Autodesk Fusion 360 part; units mm, degrees
(part 2 of 4)
sketch "intraboard_to_walls" plane through (0, 0, 0) normal (0, 0, 1) x (1, 0, 0)
  line L0 (107.12, 0) -> (107.12, 230) construction
  line L1 (100, 230) -> (-100, 230)
  line L2 (72.32, 0) -> (72.32, 230) construction
  line L3 (77.92, 0) -> (77.92, 230) construction
  line L4 (-79.68, 0) -> (-79.68, 230) construction
  line L5 (-85.28, 230) -> (-85.28, 0) construction
  line L6 (-107.12, 0) -> (-107.12, 230) construction
  line L7 (107.32, 0) -> (107.12, 0) construction
  line L8 (-107.32, 0) -> (-107.12, 0) construction
  line L9 (100, 202.925) -> (100, 197.075) construction
  line L10 (100, 157.075) -> (100, 162.925) construction
  line L11 (100, 117.075) -> (100, 122.925) construction
  line L12 (100, 77.075) -> (100, 82.925) construction
  line L13 (100, 37.075) -> (100, 42.925) construction
  line L14 (107.12, 42.925) -> (-107.12, 42.925) construction
  line L15 (107.12, 37.075) -> (-107.12, 37.075) construction
  line L16 (107.12, 77.075) -> (-107.12, 77.075) construction
  line L17 (107.12, 82.925) -> (-107.12, 82.925) construction
  line L18 (107.12, 117.075) -> (-107.12, 117.075) construction
  line L19 (107.12, 122.925) -> (-107.12, 122.925) construction
  line L20 (107.12, 157.075) -> (-107.12, 157.075) construction
  line L21 (107.12, 162.925) -> (-107.12, 162.925) construction
  line L22 (107.12, 197.075) -> (-107.12, 197.075) construction
  line L23 (107.12, 202.925) -> (-107.12, 202.925) construction
  line L24 (107.12, 208.925) -> (-107.12, 208.925) construction
  line L25 (107.12, 31.075) -> (-107.12, 31.075) construction
  line L26 (107.12, 31.075) -> (107.12, 37.075) construction
  line L27 (107.12, 202.925) -> (107.12, 208.925) construction
  line L28 (72.32, 208.925) -> (72.32, 202.925)
  line L29 (72.32, 202.925) -> (77.92, 202.925)
  line L30 (77.92, 202.925) -> (77.92, 197.075)
  line L31 (77.92, 197.075) -> (72.32, 197.075)
  line L32 (72.32, 197.075) -> (72.32, 162.925)
  line L33 (72.32, 162.925) -> (77.92, 162.925)
  line L34 (77.92, 162.925) -> (77.92, 157.075)
  line L35 (72.32, 157.075) -> (77.92, 157.075)
  line L36 (72.32, 157.075) -> (72.32, 122.925)
  line L37 (72.32, 122.925) -> (77.92, 122.925)
  line L38 (77.92, 122.925) -> (77.92, 117.075)
  line L39 (72.32, 117.075) -> (77.92, 117.075)
  line L40 (72.32, 31.075) -> (72.32, 37.075)
  line L41 (72.32, 42.925) -> (72.32, 77.075)
  line L42 (72.32, 82.925) -> (72.32, 117.075)
  line L43 (72.32, 82.925) -> (77.92, 82.925)
  line L44 (77.92, 77.075) -> (77.92, 82.925)
  line L45 (77.92, 37.075) -> (77.92, 42.925)
  line L46 (72.32, 37.075) -> (77.92, 37.075)
  line L47 (77.92, 42.925) -> (72.32, 42.925)
  line L48 (72.32, 77.075) -> (77.92, 77.075)
  line L49 (-79.68, 31.075) -> (-79.68, 37.075)
  line L50 (-79.68, 42.925) -> (-79.68, 77.075)
  line L51 (-79.68, 82.925) -> (-79.68, 117.075)
  line L52 (-79.68, 208.925) -> (-79.68, 202.925)
  line L53 (-79.68, 197.075) -> (-79.68, 162.925)
  line L54 (-79.68, 157.075) -> (-79.68, 122.925)
  line L55 (-85.28, 197.075) -> (-85.28, 202.925)
  line L56 (-85.28, 157.075) -> (-85.28, 162.925)
  line L57 (-85.28, 122.925) -> (-85.28, 117.075)
  line L58 (-85.28, 82.925) -> (-85.28, 77.075)
  line L59 (-85.28, 37.075) -> (-85.28, 42.925)
  line L60 (-79.68, 37.075) -> (-85.28, 37.075)
  line L61 (-79.68, 42.925) -> (-85.28, 42.925)
  line L62 (-79.68, 77.075) -> (-85.28, 77.075)
  line L63 (-79.68, 82.925) -> (-85.28, 82.925)
  line L64 (-79.68, 117.075) -> (-85.28, 117.075)
  line L65 (-79.68, 122.925) -> (-85.28, 122.925)
  line L66 (-79.68, 157.075) -> (-85.28, 157.075)
  line L67 (-79.68, 162.925) -> (-85.28, 162.925)
  line L68 (-85.28, 202.925) -> (-79.68, 202.925)
  line L69 (-79.68, 197.075) -> (-85.28, 197.075)
  line L70 (-107.12, 120) -> (107.12, 120) construction
  line L71 (107.12, 112.5) -> (107.12, 127.5)
  line L72 (-107.12, 112.5) -> (-107.12, 127.5)
  line L73 (-79.68, 31.075) -> (-107.12, 31.075)
  line L74 (-107.12, 31.075) -> (-107.12, 49.075)
  line L75 (-79.68, 208.925) -> (-107.12, 208.925)
  line L76 (-107.12, 208.925) -> (-107.12, 190.925)
  line L77 (72.32, 208.925) -> (107.12, 208.925)
  line L78 (107.12, 208.925) -> (107.12, 190.925)
  line L79 (72.32, 31.075) -> (107.12, 31.075)
  line L80 (107.12, 31.075) -> (107.12, 49.075)
  line L81 (-85.28, 0) -> (-90.28, 0) construction
  line L82 (-90.28, 0) -> (-90.28, 230) construction
  line L83 (77.92, 0) -> (82.92, 0) construction
  line L84 (82.92, 0) -> (82.92, 230) construction
  line L85 (-107.12, 49.075) -> (-90.28, 49.075)
  line L86 (-107.12, 112.5) -> (-90.28, 112.5)
  line L87 (-90.28, 112.5) -> (-90.28, 49.075)
  line L88 (107.12, 49.075) -> (82.92, 49.075)
  line L89 (107.12, 112.5) -> (82.92, 112.5)
  line L90 (-107.12, 190.925) -> (-90.28, 190.925)
  line L91 (107.12, 190.925) -> (82.92, 190.925)
  line L92 (107.12, 127.5) -> (82.92, 127.5)
  line L93 (-107.12, 127.5) -> (-90.28, 127.5)
  line L94 (-90.28, 127.5) -> (-90.28, 190.925)
  line L95 (82.92, 49.075) -> (82.92, 112.5)
  line L96 (82.92, 127.5) -> (82.92, 190.925)
  line L97 (-79.68, 202.925) -> (-79.68, 197.075)
  line L98 (-79.68, 162.925) -> (-79.68, 157.075)
  line L99 (-79.68, 122.925) -> (-79.68, 117.075)
  line L100 (-79.68, 82.925) -> (-79.68, 77.075)
  line L101 (-79.68, 42.925) -> (-79.68, 37.075)
  line L102 (72.32, 37.075) -> (72.32, 42.925)
  line L103 (72.32, 77.075) -> (72.32, 82.925)
  line L104 (72.32, 117.075) -> (72.32, 122.925)
  line L105 (72.32, 157.075) -> (72.32, 162.925)
  line L106 (72.32, 197.075) -> (72.32, 202.925)
  point P0 (77.92, 0)
  point P1 (72.32, 0)
  point P2 (107.32, 0)
  point P3 (-107.32, 0)
  point P4 (-85.28, 0)
  point P5 (-79.68, 0)
  point P6 (100, 40)
  point P7 (100, 80)
  point P8 (100, 120)
  point P9 (100, 160)
  point P10 (100, 200)
  point P11 (107.12, 120)
  point P12 (-107.12, 120)
  dimension "d132" = 0.2
  dimension "d133" = 5.85
  dimension "d134" = 6
  dimension "d135" = 15
  dimension "d136" = 18
  dimension "d137" = 5
  constraint coincident L0.end L1
  constraint vertical L0
  constraint horizontal P2 L0.start
  constraint coincident P1 L2.start
  constraint coincident L1 L2.end
  constraint perpendicular L1 L2
  constraint coincident P0 L3.start
  constraint coincident L1 L3.end
  constraint perpendicular L1 L3
  constraint coincident P5 L4.start
  constraint coincident L1 L4.end
  constraint perpendicular L1 L4
  constraint coincident L1 L5.start
  constraint coincident P4 L5.end
  constraint vertical L5
  constraint coincident L1 L6.end
  constraint horizontal P3 L6.start
  constraint coincident P2 L7.start
  constraint coincident P3 L8.start
  constraint equal L7 L8
  constraint vertical L6
  constraint parallel L0 L9
  constraint midpoint P10 L9
  constraint parallel L3 L10
  constraint vertical L11
  constraint vertical L12
  constraint vertical L13
  constraint equal L12 L13
  constraint equal L11 L12
  constraint equal L10 L11
  constraint equal L9 L10
  constraint midpoint P9 L10
  constraint midpoint P8 L11
  constraint midpoint P7 L12
  constraint midpoint P6 L13
  constraint coincident L0 L14.start
  constraint coincident L6 L14.end
  constraint perpendicular L6 L14
  constraint coincident L0 L15.start
  constraint coincident L6 L15.end
  constraint perpendicular L6 L15
  constraint coincident L0 L16.start
  constraint coincident L6 L16.end
  constraint perpendicular L6 L16
  constraint coincident L0 L17.start
  constraint coincident L6 L17.end
  constraint perpendicular L6 L17
  constraint coincident L0 L18.start
  constraint coincident L6 L18.end
  constraint perpendicular L6 L18
  constraint coincident L0 L19.start
  constraint coincident L6 L19.end
  constraint perpendicular L6 L19
  constraint coincident L0 L20.start
  constraint coincident L6 L20.end
  constraint perpendicular L6 L20
  constraint coincident L6 L21.end
  constraint perpendicular L6 L21
  constraint coincident L0 L22.start
  constraint coincident L6 L22.end
  constraint perpendicular L6 L22
  constraint coincident L0 L23.start
  constraint coincident L6 L23.end
  constraint perpendicular L6 L23
  constraint coincident L13.start L15
  constraint coincident L13.end L14
  constraint coincident L12.start L16
  constraint coincident L12.end L17
  constraint coincident L11.start L18
  constraint coincident L11.end L19
  constraint coincident L10.start L20
  constraint coincident L10.end L21
  constraint coincident L9.end L22
  constraint coincident L9.start L23
  constraint coincident L0 L24.start
  constraint coincident L6 L24.end
  constraint perpendicular L6 L24
  constraint coincident L6 L25.end
  constraint perpendicular L6 L25
  constraint coincident L0 L25.start
  constraint perpendicular L15 L26
  constraint equal L26 L27
  constraint coincident L24 L28.start
  constraint coincident L2 L28.start
  constraint coincident L23 L28.end
  constraint coincident L2 L28.end
  constraint coincident L23 L29.end
  constraint coincident L3 L29.end
  constraint coincident L22 L30.end
  constraint coincident L3 L30.end
  constraint coincident L2 L31.end
  constraint coincident L22 L31.end
  constraint coincident L2 L32.end
  constraint coincident L21 L32.end
  constraint coincident L3 L33.end
  constraint coincident L21 L33.end
  constraint coincident L20 L34.end
  constraint coincident L3 L34.end
  constraint coincident L20 L35.start
  constraint coincident L2 L35.start
  constraint coincident L19 L36.end
  constraint coincident L2 L36.end
  constraint coincident L19 L37.end
  constraint coincident L3 L37.end
  constraint coincident L3 L38.end
  constraint coincident L18 L38.end
  constraint coincident L18 L39.start
  constraint perpendicular L38 L39
  constraint coincident L25 L40.start
  constraint coincident L2 L40.start
  constraint coincident L15 L40.end
  constraint coincident L2 L40.end
  constraint coincident L14 L41.start
  constraint coincident L2 L41.start
  constraint coincident L16 L41.end
  constraint coincident L2 L41.end
  constraint coincident L17 L42.start
  constraint coincident L2 L42.start
  constraint perpendicular L18 L42
  constraint coincident L17 L43.end
  constraint coincident L3 L43.end
  constraint coincident L16 L44.start
  constraint coincident L3 L44.start
  constraint coincident L15 L45.start
  constraint coincident L3 L45.start
  constraint coincident L14 L45.end
  constraint coincident L3 L45.end
  constraint coincident L4 L49.start
  constraint coincident L25 L49.start
  constraint coincident L15 L49.end
  constraint coincident L4 L49.end
  constraint coincident L14 L50.start
  constraint coincident L4 L50.start
  constraint coincident L4 L50.end
  constraint coincident L16 L50.end
  constraint coincident L4 L51.start
  constraint coincident L17 L51.start
  constraint coincident L4 L51.end
  constraint coincident L18 L51.end
  constraint coincident L24 L52.start
  constraint coincident L4 L52.start
  constraint coincident L4 L52.end
  constraint coincident L23 L52.end
  constraint coincident L4 L53.start
  constraint coincident L22 L53.start
  constraint coincident L4 L53.end
  constraint coincident L21 L53.end
  constraint coincident L20 L54.start
  constraint coincident L4 L54.start
  constraint coincident L19 L54.end
  constraint coincident L4 L54.end
  constraint coincident L22 L55.start
  constraint coincident L5 L55.start
  constraint coincident L23 L55.end
  constraint coincident L5 L55.end
  constraint coincident L20 L56.start
  constraint coincident L5 L56.start
  constraint coincident L21 L56.end
  constraint coincident L5 L56.end
  constraint coincident L19 L57.start
  constraint coincident L5 L57.start
  constraint coincident L5 L57.end
  constraint coincident L18 L57.end
  constraint coincident L17 L58.start
  constraint coincident L5 L58.start
  constraint coincident L16 L58.end
  constraint coincident L5 L58.end
  constraint coincident L15 L59.start
  constraint coincident L5 L59.start
  constraint coincident L14 L59.end
  constraint coincident L5 L59.end
  constraint coincident L0 P11
  constraint coincident L6 P12
  constraint coincident P12 L70.start
  constraint coincident P11 L70.end
  constraint horizontal L70
  constraint coincident P8 L70
  constraint perpendicular L70 L71
  constraint midpoint P11 L71
  constraint coincident L0 L21.start
  constraint parallel L6 L72
  constraint equal L71 L72
  constraint midpoint P12 L72
  constraint coincident L6 L74.end
  constraint coincident L6 L76.end
  constraint coincident L0 L78.end
  constraint coincident L0 L80.end
  constraint equal L74 L80
  constraint equal L74 L76
  constraint equal L78 L80
  constraint perpendicular L5 L81
  constraint coincident L1 L82.end
  constraint perpendicular L1 L82
  constraint perpendicular L3 L83
  constraint coincident L1 L84.end
  constraint perpendicular L1 L84
  constraint equal L81 L83
  constraint coincident L82 L85.end
  constraint perpendicular L82 L85
  constraint coincident L82 L86.end
  constraint perpendicular L82 L86
  constraint coincident L84 L88.end
  constraint perpendicular L84 L88
  constraint coincident L84 L89.end
  constraint perpendicular L84 L89
  constraint coincident L82 L90.end
  constraint perpendicular L82 L90
  constraint coincident L84 L91.end
  constraint perpendicular L84 L91
  constraint coincident L84 L92.end
  constraint perpendicular L84 L92
  constraint coincident L82 L93.end
  constraint perpendicular L82 L93
  measures "d132" distance of P2 L0
  measures "d133" distance of L9.start L9.end
  measures "d134" distance of L15.start L25.start
  measures "d135" distance of L71.start L71.end
  measures "d136" distance of L25.end L74.end
  measures "d137" distance of P4 L81.end
extrude "Extrude5" add sketch "intraboard_to_walls" along normal up to surface (25.6 mm away) from surface at 21.5 separate body contours L28 L29 L30 L31 L32 L33 L34 L35 L36 L37 L38 L39 L40 L41 L42 L43 L44 L45 L46 L47 L48 L71 L77 L78 L79 L80 L88 L89 L91 L92 L95 L96 makes body 7
extrude "Extrude6" add sketch "intraboard_to_walls" along normal up to surface (5 mm away) from surface at 42.1 contours L29 L30 L31 L106 | L33 L34 L35 L105 | L37 L38 L39 L104 | L43 L44 L48 L103 | L45 L46 L47 L102 bodies 7
extrude "Extrude7" add sketch "intraboard_to_walls" along normal up to surface (22.6 mm away) from surface at 21.5 separate body contours L49 L50 L51 L52 L53 L54 L55 L56 L57 L58 L59 L60 L61 L62 L63 L64 L65 L66 L67 L68 L69 L72 L73 L74 L75 L76 L85 L86 L87 L90 L93 L94 makes body 8
extrude "Extrude8" add sketch "intraboard_to_walls" along normal up to surface (2 mm away) from surface at 42.1 contours L59 L60 L61 L101 | L58 L62 L63 L100 | L57 L64 L65 L99 | L56 L66 L67 L98 | L55 L68 L69 L97 bodies 8
extrude "Extrude9" add sketch "left side panel" along normal up to surface (5.36 mm away) from surface at 107.32 separate body makes body 9
ref_plane "WorkPlane1" through (-107.32, 0, 0) normal (1, 0, 0) x (0, 1, 0)
sketch "right side panel" plane through (-107.32, 0, 0) normal (1, 0, 0) x (0, 0, -1)
  line L0 (-105.5, 215.5) -> (105.5, 215.5)
  line L1 (105.5, 215.5) -> (105.5, 4.5)
  line L2 (-105.5, 4.5) -> (-105.5, 215.5)
  line L3 (105.5, 4.5) -> (-105.5, 4.5)
  line L4 (-21.5, 31.075) -> (-44.1, 31.075)
  line L5 (-44.1, 31.075) -> (-44.1, 49.075)
  line L6 (-44.1, 49.075) -> (-21.5, 49.075)
  line L7 (-21.5, 49.075) -> (-21.5, 31.075)
  line L8 (-21.5, 127.5) -> (-44.1, 127.5)
  line L9 (-44.1, 127.5) -> (-44.1, 112.5)
  line L10 (-44.1, 112.5) -> (-21.5, 112.5)
  line L11 (-21.5, 112.5) -> (-21.5, 127.5)
  line L12 (-21.5, 208.925) -> (-44.1, 208.925)
  line L13 (-44.1, 208.925) -> (-44.1, 190.925)
  line L14 (-44.1, 190.925) -> (-21.5, 190.925)
  line L15 (-21.5, 190.925) -> (-21.5, 208.925)
  line L16 (105.5, 215.5) -> (100, 215.5) construction
  line L17 (100, 215.5) -> (100, 210) construction
  line L18 (100, 210) -> (105.5, 210) construction
  line L19 (105.5, 210) -> (105.5, 215.5) construction
  line L20 (-105.5, 4.5) -> (-100, 4.5) construction
  line L21 (-100, 4.5) -> (-100, 10) construction
  line L22 (-100, 10) -> (-105.5, 10) construction
  line L23 (-105.5, 10) -> (-105.5, 4.5) construction
  line L24 (100, 210) -> (-100, 210) construction
  line L25 (-100, 210) -> (-100, 10) construction
  line L26 (-100, 10) -> (100, 10) construction
  line L27 (100, 10) -> (100, 210) construction
  line L28 (-100, 10) -> (-85, 10) construction
  line L29 (-85, 10) -> (-85, 25) construction
  line L30 (-85, 25) -> (-100, 25) construction
  line L31 (-100, 25) -> (-100, 10) construction
  line L32 (-73, 25) -> (-79, 35.3923) construction
  line L33 (-79, 35.3923) -> (-85, 25) construction
  line L34 (-85, 25) -> (-73, 25) construction
  line L35 (-79, 35.3923) -> (-73, 45.7846) construction
  line L36 (-73, 45.7846) -> (-85, 45.7846) construction
  line L37 (-85, 45.7846) -> (-79, 35.3923) construction
  line L38 (-100, 10) -> (-95, 10) construction
  line L39 (-95, 10) -> (-95, 15) construction
  line L40 (-95, 15) -> (-100, 15) construction
  line L41 (-100, 15) -> (-100, 10) construction
  line L42 (-100, 210) -> (-95, 210) construction
  line L43 (-95, 210) -> (-95, 205) construction
  line L44 (-95, 205) -> (-100, 205) construction
  line L45 (-100, 205) -> (-100, 210) construction
  line L46 (-95, 15) -> (-15, 15) construction
  line L47 (-15, 15) -> (-15, 205) construction
  line L48 (-15, 205) -> (-95, 205) construction
  line L49 (-95, 205) -> (-95, 15) construction
  line L50 (-79, 35.3923) -> (-91, 35.3923) construction
  line L51 (-21.5, 208.925) -> (-44.1, 190.925) construction
  line L52 (-21.5, 127.5) -> (-44.1, 112.5) construction
  line L53 (-21.5, 49.075) -> (-44.1, 31.075) construction
  arc A0 (-32.4011, 44.6367) -> (-33.1989, 44.6367) centre (-32.8, 44.667) ccw
  line L54 (-32.8, 40.075) -> (-32.8, 44.867) construction
  line L55 (-36.95, 42.0104) -> (-36.95, 38.1396)
  line L56 (-36.5511, 37.4487) -> (-33.1989, 35.5133)
  line L57 (-28.65, 38.1396) -> (-28.65, 42.0104)
  arc A1 (-33.1989, 35.5133) -> (-32.4011, 35.5133) centre (-32.8, 35.483) ccw
  line L58 (-28.65, 37.679) -> (-28.65, 42.471) construction
  line L59 (-32.4011, 35.5133) -> (-29.0489, 37.4487)
  arc A2 (-28.65, 42.0104) -> (-29.0489, 42.7013) centre (-28.8232, 42.371) ccw
  line L60 (-36.95, 42.471) -> (-36.95, 37.679) construction
  line L61 (-28.65, 42.471) -> (-32.8, 44.867) construction
  circle A3 centre (-32.8, 44.667) radius 0.4 construction
  line L62 (-33.1989, 44.6367) -> (-36.5511, 42.7013)
  line L63 (-29.0489, 42.7013) -> (-32.4011, 44.6367)
  arc A4 (-36.95, 38.1396) -> (-36.5511, 37.4487) centre (-36.7768, 37.779) ccw
  line L64 (-32.8, 44.867) -> (-36.95, 42.471) construction
  arc A5 (-36.5511, 42.7013) -> (-36.95, 42.0104) centre (-36.7768, 42.371) ccw
  line L65 (-36.95, 37.679) -> (-32.8, 35.283) construction
  line L66 (-32.8, 35.283) -> (-28.65, 37.679) construction
  arc A6 (-29.0489, 37.4487) -> (-28.65, 38.1396) centre (-28.8232, 37.779) ccw
  arc A7 (-33.1989, 115.4383) -> (-32.4011, 115.4383) centre (-32.8, 115.408) ccw
  arc A8 (-32.4011, 124.5617) -> (-33.1989, 124.5617) centre (-32.8, 124.592) ccw
  line L67 (-29.0489, 122.6263) -> (-32.4011, 124.5617)
  line L68 (-28.65, 122.396) -> (-32.8, 124.792) construction
  line L69 (-28.65, 117.604) -> (-28.65, 122.396) construction
  line L70 (-32.8, 124.792) -> (-36.95, 122.396) construction
  line L71 (-32.8, 115.208) -> (-28.65, 117.604) construction
  line L72 (-33.1989, 124.5617) -> (-36.5511, 122.6263)
  line L73 (-32.8, 120) -> (-32.8, 124.792) construction
  line L74 (-36.95, 117.604) -> (-32.8, 115.208) construction
  line L75 (-32.4011, 115.4383) -> (-29.0489, 117.3737)
  line L76 (-28.65, 118.0646) -> (-28.65, 121.9354)
  arc A9 (-28.65, 121.9354) -> (-29.0489, 122.6263) centre (-28.8232, 122.296) ccw
  arc A10 (-36.5511, 122.6263) -> (-36.95, 121.9354) centre (-36.7768, 122.296) ccw
  line L77 (-36.95, 122.396) -> (-36.95, 117.604) construction
  circle A11 centre (-32.8, 124.592) radius 0.4 construction
  arc A12 (-29.0489, 117.3737) -> (-28.65, 118.0646) centre (-28.8232, 117.704) ccw
  line L78 (-36.95, 121.9354) -> (-36.95, 118.0646)
  arc A13 (-36.95, 118.0646) -> (-36.5511, 117.3737) centre (-36.7768, 117.704) ccw
  line L79 (-36.5511, 117.3737) -> (-33.1989, 115.4383)
  arc A14 (-33.1989, 195.3633) -> (-32.4011, 195.3633) centre (-32.8, 195.333) ccw
  arc A15 (-32.4011, 204.4867) -> (-33.1989, 204.4867) centre (-32.8, 204.517) ccw
  line L80 (-29.0489, 202.5513) -> (-32.4011, 204.4867)
  line L81 (-28.65, 202.321) -> (-32.8, 204.717) construction
  line L82 (-28.65, 197.529) -> (-28.65, 202.321) construction
  line L83 (-32.8, 204.717) -> (-36.95, 202.321) construction
  line L84 (-32.8, 195.133) -> (-28.65, 197.529) construction
  line L85 (-33.1989, 204.4867) -> (-36.5511, 202.5513)
  line L86 (-32.8, 199.925) -> (-32.8, 204.717) construction
  line L87 (-36.95, 197.529) -> (-32.8, 195.133) construction
  line L88 (-32.4011, 195.3633) -> (-29.0489, 197.2987)
  line L89 (-28.65, 197.9896) -> (-28.65, 201.8604)
  arc A16 (-28.65, 201.8604) -> (-29.0489, 202.5513) centre (-28.8232, 202.221) ccw
  arc A17 (-36.5511, 202.5513) -> (-36.95, 201.8604) centre (-36.7768, 202.221) ccw
  line L90 (-36.95, 202.321) -> (-36.95, 197.529) construction
  circle A18 centre (-32.8, 204.517) radius 0.4 construction
  arc A19 (-29.0489, 197.2987) -> (-28.65, 197.9896) centre (-28.8232, 197.629) ccw
  line L91 (-36.95, 201.8604) -> (-36.95, 197.9896)
  arc A20 (-36.95, 197.9896) -> (-36.5511, 197.2987) centre (-36.7768, 197.629) ccw
  line L92 (-36.5511, 197.2987) -> (-33.1989, 195.3633)
  point P0 (-21.5, 0)
  point P1 (-44.1, 0)
  point P2 (0, 31.075)
  point P3 (0, 49.075)
  point P4 (0, 112.5)
  point P5 (0, 127.5)
  point P6 (0, 190.925)
  point P7 (0, 208.925)
  point P8 (-79, 28.4641)
  point P9 (-61, 25)
  point P10 (-49, 25)
  point P11 (-37, 25)
  point P12 (-25, 25)
  point P13 (-85, 45.785)
  point P14 (-73, 45.785)
  point P15 (-61, 45.785)
  point P16 (-49, 45.785)
  point P17 (-85, 66.57)
  point P18 (-73, 66.57)
  point P19 (-61, 66.57)
  point P20 (-49, 66.57)
  point P21 (-37, 66.57)
  point P22 (-25, 66.57)
  point P23 (-85, 87.355)
  point P24 (-73, 87.355)
  point P25 (-61, 87.355)
  point P26 (-49, 87.355)
  point P27 (-37, 87.355)
  point P28 (-25, 87.355)
  point P29 (-85, 108.14)
  point P30 (-73, 108.14)
  point P31 (-61, 108.14)
  point P32 (-49, 108.14)
  point P33 (-85, 128.925)
  point P34 (-73, 128.925)
  point P35 (-61, 128.925)
  point P36 (-49, 128.925)
  point P37 (-85, 149.71)
  point P38 (-73, 149.71)
  point P39 (-61, 149.71)
  point P40 (-49, 149.71)
  point P41 (-37, 149.71)
  point P42 (-25, 149.71)
  point P43 (-85, 170.495)
  point P44 (-73, 170.495)
  point P45 (-61, 170.495)
  point P46 (-49, 170.495)
  point P47 (-37, 170.495)
  point P48 (-25, 170.495)
  point P49 (-85, 191.28)
  point P50 (-73, 191.28)
  point P51 (-61, 191.28)
  point P52 (-49, 191.28)
  point P53 (-67, 35.3923)
  point P54 (-55, 35.3923)
  point P55 (-91, 56.1773)
  point P56 (-79, 56.1773)
  point P57 (-67, 56.1773)
  point P58 (-55, 56.1773)
  point P59 (-43, 56.1773)
  point P60 (-31, 56.1773)
  point P61 (-19, 56.1773)
  point P62 (-91, 76.9623)
  point P63 (-79, 76.9623)
  point P64 (-67, 76.9623)
  point P65 (-55, 76.9623)
  point P66 (-43, 76.9623)
  point P67 (-31, 76.9623)
  point P68 (-19, 76.9623)
  point P69 (-91, 97.7473)
  point P70 (-79, 97.7473)
  point P71 (-67, 97.7473)
  point P72 (-55, 97.7473)
  point P73 (-43, 97.7473)
  point P74 (-31, 97.7473)
  point P75 (-19, 97.7473)
  point P76 (-91, 118.5323)
  point P77 (-79, 118.5323)
  point P78 (-67, 118.5323)
  point P79 (-55, 118.5323)
  point P80 (-91, 139.3173)
  point P81 (-79, 139.3173)
  point P82 (-67, 139.3173)
  point P83 (-55, 139.3173)
  point P84 (-43, 139.3173)
  point P85 (-31, 139.3173)
  point P86 (-19, 139.3173)
  point P87 (-91, 160.1023)
  point P88 (-79, 160.1023)
  point P89 (-67, 160.1023)
  point P90 (-55, 160.1023)
  point P91 (-43, 160.1023)
  point P92 (-31, 160.1023)
  point P93 (-19, 160.1023)
  point P94 (-91, 180.8873)
  point P95 (-79, 180.8873)
  point P96 (-67, 180.8873)
  point P97 (-55, 180.8873)
  point P98 (-43, 180.8873)
  point P99 (-31, 180.8873)
  point P100 (-19, 180.8873)
  point P101 (-91, 201.6723)
  point P102 (-79, 201.6723)
  point P103 (-67, 201.6723)
  point P104 (-55, 201.6723)
  point P105 (-32.8, 40.075)
  point P106 (-32.8, 120)
  point P107 (-32.8, 199.925)
  point P108 (-32.8, 40.075)
  point P109 (-32.8, 40.075)
  point P110 (-32.8, 40.075)
  point P111 (-32.8, 40.075)
  point P112 (-32.8, 120)
  point P113 (-32.8, 120)
  point P114 (-32.8, 120)
  point P115 (-32.8, 120)
  point P116 (-32.8, 120)
  point P117 (-32.8, 199.925)
  point P118 (-32.8, 199.925)
  point P119 (-32.8, 199.925)
  point P120 (-32.8, 199.925)
  point P121 (-32.8, 199.925)
  dimension "d154" = 5.5
  dimension "d156" = 15
  dimension "d157" = 15
  dimension "d158" = 12
  dimension "d159" = 12
  dimension "d160" = 20.7846
  dimension "d161" = 5
  dimension "d162" = 5
  dimension "d163" = 80
  dimension "d166" = 12
  dimension "d167" = 20.785
  dimension "d171" = 12
  dimension "d172" = 20.785
  dimension "d261" = 360
  dimension "d263" = 360
  dimension "d264" = 4.15
  dimension "d265" = 0.8
  dimension "d266" = 0.2
  dimension "d268" = 360
  dimension "d270" = 360
  dimension "d271" = 4.15
  dimension "d272" = 0.8
  dimension "d273" = 0.2
  dimension "d275" = 360
  dimension "d277" = 360
  dimension "d278" = 4.15
  dimension "d279" = 0.8
  dimension "d280" = 0.2
  constraint horizontal L4
  constraint vertical L5
  constraint horizontal L6
  constraint vertical L7
  constraint horizontal L8
  constraint vertical L9
  constraint horizontal L10
  constraint vertical L11
  constraint horizontal L12
  constraint vertical L13
  constraint horizontal L14
  constraint vertical L15
  constraint coincident P7 L12
  constraint coincident P6 L14
  constraint coincident P5 L8
  constraint coincident P4 L10
  constraint coincident P3 L6
  constraint coincident P2 L4
  constraint coincident P0 L7
  constraint coincident P1 L5
  constraint coincident P0 L11
  constraint coincident P1 L9
  constraint coincident P0 L15
  constraint coincident P1 L13
  constraint horizontal L16
  constraint vertical L17
  constraint horizontal L18
  constraint vertical L19
  constraint coincident L0.end L1.start
  constraint equal L17 L18
  constraint horizontal L20
  constraint vertical L21
  constraint horizontal L22
  constraint vertical L23
  constraint coincident L2.start L3.end
  constraint equal L21 L22
  constraint equal L18 L22
  constraint horizontal L24
  constraint vertical L25
  constraint horizontal L26
  constraint vertical L27
  constraint horizontal L28
  constraint vertical L29
  constraint horizontal L30
  constraint vertical L31
  constraint coincident L29.end L30.start
  constraint horizontal L34
  constraint parallel L33 L35
  constraint horizontal L36
  constraint parallel L32 L37
  constraint horizontal L38
  constraint vertical L39
  constraint horizontal L40
  constraint vertical L41
  constraint horizontal L42
  constraint vertical L43
  constraint horizontal L44
  constraint vertical L45
  constraint equal L43 L44
  constraint equal L40 L44
  constraint horizontal L46
  constraint vertical L47
  constraint horizontal L48
  constraint vertical L49
  constraint coincident L43.end L44.start
  constraint horizontal L50
  constraint equal L34 L50
  constraint midpoint L53 P111
  constraint midpoint L52 P116
  constraint midpoint L51 P121
  constraint coincident P111 P110
  constraint vertical L60
  constraint coincident A0.centre L54
  constraint coincident A0.end L64
  constraint coincident A0.start L61
  constraint coincident A0.start A3
  constraint coincident A0.centre A3.centre
  constraint coincident P116 P115
  constraint vertical L77
  constraint coincident A8.centre L73
  constraint coincident A8.end L70
  constraint coincident A8.start L68
  constraint coincident A8.start A11
  constraint coincident A8.centre A11.centre
  constraint coincident P121 P120
  constraint vertical L90
  constraint coincident A15.centre L86
  constraint coincident A15.end L83
  constraint coincident A15.start L81
  constraint coincident A15.start A18
  constraint coincident A15.centre A18.centre
  measures "d154" distance of L0.end L18.end
  measures "d156" distance of L21.end L28.end
  measures "d157" distance of L21.end L30.end
  measures "d158" distance of L32.start L29.end
  measures "d159" distance of L32.end L35.end
  measures "d160" distance of L29.end L36.end
  measures "d161" distance of L21.end L38.end
  measures "d162" distance of L21.end L40.end
  measures "d163" distance of L39.end L46.end
  measures "d264" distance of P111 L60
  measures "d265" diameter of A3
  measures "d266" distance of L54.end A0.centre
  measures "d271" distance of P116 L77
  measures "d272" diameter of A11
  measures "d273" distance of A8.centre L68.end
  measures "d278" distance of P121 L90
  measures "d279" diameter of A18
  measures "d280" distance of A15.centre L81.end
extrude "Extrude10" add sketch "right side panel" against normal up to surface (5.36 mm away) separate body contours L0 L1 L2 L3 | L4 L5 L6 L7 | L8 L9 L10 L11 | L12 L13 L14 L15 | A0 L55 L56 L57 A1 L59 A2 L62 L63 A4 A5 A6 | A7 A8 L67 L72 L75 L76 A9 A10 A12 L78 A13 L79 | A14 A15 L80 L85 L88 L89 A16 A17 A19 L91 A20 L92 makes body 10
hole "Hole1" at (-107.32, 191.28, 61) at (-107.32, 191.28, 49) at (-107.32, 180.8873, 43) at (-107.32, 180.8873, 31) at (-107.32, 180.8873, 19) at (-107.32, 170.495, 25) at (-107.32, 160.1023, 19) at (-107.32, 149.71, 25) at (-107.32, 139.3173, 19) at (-107.32, 139.3173, 31) at (-107.32, 139.3173, 43) at (-107.32, 128.925, 49) at (-107.32, 118.5323, 55) at (-107.32, 108.14, 49) at (-107.32, 97.7473, 43) at (-107.32, 97.7473, 31) at (-107.32, 97.7473, 19) at (-107.32, 87.355, 25) at (-107.32, 87.355, 37) at (-107.32, 76.9623, 19) at (-107.32, 76.9623, 31) at (-107.32, 76.9623, 43) at (-107.32, 87.355, 49) at (-107.32, 56.1773, 19) at (-107.32, 66.57, 25) at (-107.32, 56.1773, 31) at (-107.32, 56.1773, 43) at (-107.32, 45.785, 49) at (-107.32, 35.3923, 55) at (-107.32, 25, 49) at (-107.32, 25, 37) at (-107.32, 25, 25) at (-107.32, 25, 61) at (-107.32, 35.3923, 67) at (-107.32, 45.785, 61) at (-107.32, 25, 73) at (-107.32, 25, 85) at (-107.32, 35.3923, 79) at (-107.32, 45.785, 85) at (-107.32, 45.785, 73) at (-107.32, 56.1773, 67) at (-107.32, 56.1773, 55) at (-107.32, 66.57, 49) at (-107.32, 66.57, 37) at (-107.32, 66.57, 61) at (-107.32, 76.9623, 55) at (-107.32, 76.9623, 67) at (-107.32, 66.57, 73) at (-107.32, 87.355, 61) at (-107.32, 56.1773, 79) at (-107.32, 66.57, 85) at (-107.32, 76.9623, 79) at (-107.32, 87.355, 85) at (-107.32, 87.355, 73) at (-107.32, 97.7473, 79) at (-107.32, 108.14, 85) at (-107.32, 118.5323, 79) at (-107.32, 128.925, 85) at (-107.32, 139.3173, 79) at (-107.32, 149.71, 85) at (-107.32, 160.1023, 79) at (-107.32, 160.1023, 67) at (-107.32, 160.1023, 55) at (-107.32, 160.1023, 43) at (-107.32, 160.1023, 31) at (-107.32, 149.71, 37) at (-107.32, 149.71, 49) at (-107.32, 149.71, 61) at (-107.32, 139.3173, 55) at (-107.32, 128.925, 61) at (-107.32, 108.14, 61) at (-107.32, 97.7473, 55) at (-107.32, 97.7473, 67) at (-107.32, 108.14, 73) at (-107.32, 118.5323, 67) at (-107.32, 128.925, 73) at (-107.32, 139.3173, 67) at (-107.32, 149.71, 73) at (-107.32, 170.495, 85) at (-107.32, 180.8873, 79) at (-107.32, 191.28, 85) at (-107.32, 191.28, 73) at (-107.32, 180.8873, 67) at (-107.32, 180.8873, 55) at (-107.32, 170.495, 37) at (-107.32, 170.495, 49) at (-107.32, 170.495, 61) at (-107.32, 170.495, 73) direction (-1, 0, 0) diameter 10 end up to surface (5.36 mm away) bodies 10
sketch "left_side_misc" plane through (0, 0, 0) normal (1, 0, 0) x (0, 0, -1)
  line L0 (-47.1, 208.925) -> (-47.1, 190.925) construction
  line L1 (-47.1, 190.925) -> (-21.5, 190.925) construction
  line L2 (-21.5, 190.925) -> (-21.5, 208.925) construction
  line L3 (-21.5, 208.925) -> (-47.1, 208.925) construction
  line L4 (-47.1, 127.5) -> (-47.1, 112.5) construction
  line L5 (-47.1, 112.5) -> (-21.5, 112.5) construction
  line L6 (-21.5, 112.5) -> (-21.5, 127.5) construction
  line L7 (-21.5, 127.5) -> (-47.1, 127.5) construction
  line L8 (-47.1, 49.075) -> (-47.1, 31.075) construction
  line L9 (-47.1, 31.075) -> (-21.5, 31.075) construction
  line L10 (-21.5, 31.075) -> (-21.5, 49.075) construction
  line L11 (-21.5, 49.075) -> (-47.1, 49.075) construction
  line L12 (-47.1, 208.925) -> (-21.5, 190.925) construction
  line L13 (-47.1, 127.5) -> (-21.5, 112.5) construction
  line L14 (-21.5, 31.075) -> (-47.1, 49.075) construction
  line L15 (-77, 45) -> (-51, 45)
  line L16 (-51, 45) -> (-51, 14)
  line L17 (-51, 14) -> (-77, 14)
  line L18 (-77, 14) -> (-77, 45)
  line L19 (-64, 14) -> (-64, 45) construction
  line L20 (-51, 29.5) -> (-77, 29.5) construction
  line L21 (-73.6, 41.5) -> (-54.4, 17.5) construction
  circle A0 centre (-64, 29.5) radius 11.6
  circle A1 centre (-73.6, 41.5) radius 1.1
  circle A2 centre (-54.4, 17.5) radius 1.1
  line L22 (-30.15, 122.396) -> (-34.3, 124.792) construction
  line L23 (-34.3, 124.792) -> (-38.45, 122.396) construction
  line L24 (-38.45, 122.396) -> (-38.45, 117.604) construction
  line L25 (-38.45, 117.604) -> (-34.3, 115.208) construction
  line L26 (-34.3, 115.208) -> (-30.15, 117.604) construction
  line L27 (-30.15, 117.604) -> (-30.15, 122.396) construction
  circle A3 centre (-34.3, 124.592) radius 0.4 construction
  circle A4 centre (-38.2768, 122.296) radius 0.4 construction
  circle A5 centre (-38.2768, 117.704) radius 0.4 construction
  circle A6 centre (-34.3, 115.408) radius 0.4 construction
  circle A7 centre (-30.3232, 117.704) radius 0.4 construction
  circle A8 centre (-30.3232, 122.296) radius 0.4 construction
  arc A9 (-33.9011, 124.5617) -> (-34.6989, 124.5617) centre (-34.3, 124.592) ccw
  arc A10 (-38.0511, 122.6263) -> (-38.45, 121.9354) centre (-38.2768, 122.296) ccw
  arc A11 (-38.45, 118.0646) -> (-38.0511, 117.3737) centre (-38.2768, 117.704) ccw
  arc A12 (-34.6989, 115.4383) -> (-33.9011, 115.4383) centre (-34.3, 115.408) ccw
  arc A13 (-30.5489, 117.3737) -> (-30.15, 118.0646) centre (-30.3232, 117.704) ccw
  arc A14 (-30.15, 121.9354) -> (-30.5489, 122.6263) centre (-30.3232, 122.296) ccw
  line L28 (-33.9011, 124.5617) -> (-30.5489, 122.6263)
  line L29 (-38.0511, 122.6263) -> (-34.6989, 124.5617)
  line L30 (-38.45, 118.0646) -> (-38.45, 121.9354)
  line L31 (-34.6989, 115.4383) -> (-38.0511, 117.3737)
  line L32 (-30.5489, 117.3737) -> (-33.9011, 115.4383)
  line L33 (-30.15, 121.9354) -> (-30.15, 118.0646)
  line L34 (-30.5489, 37.4487) -> (-33.9011, 35.5133)
  arc A15 (-30.5489, 37.4487) -> (-30.15, 38.1396) centre (-30.3232, 37.779) ccw
  circle A16 centre (-38.2768, 42.371) radius 0.4 construction
  arc A17 (-30.15, 42.0104) -> (-30.5489, 42.7013) centre (-30.3232, 42.371) ccw
  circle A18 centre (-38.2768, 37.779) radius 0.4 construction
  line L35 (-34.6989, 35.5133) -> (-38.0511, 37.4487)
  arc A19 (-38.45, 38.1396) -> (-38.0511, 37.4487) centre (-38.2768, 37.779) ccw
  line L36 (-34.3, 44.867) -> (-38.45, 42.471) construction
  circle A20 centre (-34.3, 44.667) radius 0.4 construction
  line L37 (-38.45, 38.1396) -> (-38.45, 42.0104)
  circle A21 centre (-30.3232, 37.779) radius 0.4 construction
  line L38 (-30.15, 42.471) -> (-34.3, 44.867) construction
  circle A22 centre (-30.3232, 42.371) radius 0.4 construction
  arc A23 (-38.0511, 42.7013) -> (-38.45, 42.0104) centre (-38.2768, 42.371) ccw
  line L39 (-30.15, 42.0104) -> (-30.15, 38.1396)
  line L40 (-38.45, 42.471) -> (-38.45, 37.679) construction
  circle A24 centre (-34.3, 35.483) radius 0.4 construction
  arc A25 (-34.6989, 35.5133) -> (-33.9011, 35.5133) centre (-34.3, 35.483) ccw
  line L41 (-38.45, 37.679) -> (-34.3, 35.283) construction
  line L42 (-30.15, 37.679) -> (-30.15, 42.471) construction
  line L43 (-38.0511, 42.7013) -> (-34.6989, 44.6367)
  line L44 (-33.9011, 44.6367) -> (-30.5489, 42.7013)
  line L45 (-34.3, 35.283) -> (-30.15, 37.679) construction
  arc A26 (-33.9011, 44.6367) -> (-34.6989, 44.6367) centre (-34.3, 44.667) ccw
  line L46 (-30.5489, 197.2987) -> (-33.9011, 195.3633)
  arc A27 (-30.5489, 197.2987) -> (-30.15, 197.9896) centre (-30.3232, 197.629) ccw
  circle A28 centre (-38.2768, 202.221) radius 0.4 construction
  arc A29 (-30.15, 201.8604) -> (-30.5489, 202.5513) centre (-30.3232, 202.221) ccw
  circle A30 centre (-38.2768, 197.629) radius 0.4 construction
  line L47 (-34.6989, 195.3633) -> (-38.0511, 197.2987)
  arc A31 (-38.45, 197.9896) -> (-38.0511, 197.2987) centre (-38.2768, 197.629) ccw
  line L48 (-34.3, 204.717) -> (-38.45, 202.321) construction
  circle A32 centre (-34.3, 204.517) radius 0.4 construction
  line L49 (-38.45, 197.9896) -> (-38.45, 201.8604)
  circle A33 centre (-30.3232, 197.629) radius 0.4 construction
  line L50 (-30.15, 202.321) -> (-34.3, 204.717) construction
  circle A34 centre (-30.3232, 202.221) radius 0.4 construction
  arc A35 (-38.0511, 202.5513) -> (-38.45, 201.8604) centre (-38.2768, 202.221) ccw
  line L51 (-30.15, 201.8604) -> (-30.15, 197.9896)
  line L52 (-38.45, 202.321) -> (-38.45, 197.529) construction
  circle A36 centre (-34.3, 195.333) radius 0.4 construction
  arc A37 (-34.6989, 195.3633) -> (-33.9011, 195.3633) centre (-34.3, 195.333) ccw
  line L53 (-38.45, 197.529) -> (-34.3, 195.133) construction
  line L54 (-30.15, 197.529) -> (-30.15, 202.321) construction
  line L55 (-38.0511, 202.5513) -> (-34.6989, 204.4867)
  line L56 (-33.9011, 204.4867) -> (-30.5489, 202.5513)
  line L57 (-34.3, 195.133) -> (-30.15, 197.529) construction
  arc A38 (-33.9011, 204.4867) -> (-34.6989, 204.4867) centre (-34.3, 204.517) ccw
  line L58 (-73.6, 41.5) -> (-54.4, 41.5) construction
  line L59 (-54.4, 41.5) -> (-54.4, 17.5) construction
  line L60 (-54.4, 17.5) -> (-73.6, 17.5) construction
  line L61 (-73.6, 17.5) -> (-73.6, 41.5) construction
  point P0 (-34.3, 199.925)
  point P1 (-34.3, 120)
  point P2 (-34.3, 40.075)
  point P3 (-100, 10)
  point P4 (-64, 29.5)
  point P5 (-34.3, 120)
  point P6 (-34.3, 40.075)
  point P7 (-34.3, 40.075)
  point P8 (-34.3, 199.925)
  point P9 (-34.3, 199.925)
  dimension "d221" = 26
  dimension "d222" = 31
  dimension "d223" = 4
  dimension "d224" = 23
  dimension "d227" = 23.2
  dimension "d228" = 2.2
  dimension "d232" = 4.15
  dimension "d233" = 0.8
  dimension "d235" = 0.2
  dimension "d237" = 360
  dimension "d239" = 360
  dimension "d241" = 360
  dimension "d243" = 360
  dimension "d245" = 360
  dimension "d247" = 360
  dimension "d248" = 4.15
  dimension "d249" = 0.8
  dimension "d250" = 0.2
  dimension "d252" = 360
  dimension "d254" = 360
  dimension "d256" = 360
  dimension "d257" = 4.15
  dimension "d258" = 0.8
  dimension "d259" = 0.2
  dimension "d342" = 24
  dimension "d343" = 19.2
  constraint coincident L0.start L3.end
  constraint coincident L1.end L2.start
  constraint coincident L4.start L7.end
  constraint coincident L5.end L6.start
  constraint coincident L9.end L10.start
  constraint coincident L8.start L11.end
  constraint midpoint L12 P9
  constraint midpoint L13 P5
  constraint midpoint L14 P7
  constraint horizontal L15
  constraint vertical L16
  constraint horizontal L17
  constraint vertical L18
  constraint midpoint L17 L19.start
  constraint midpoint L15 L19.end
  constraint midpoint L16 L20.start
  constraint midpoint L18 L20.end
  constraint coincident L21 P4
  constraint midpoint L20 P4
  constraint coincident P4 A0.centre
  constraint coincident L21.start A1.centre
  constraint coincident L21.end A2.centre
  constraint equal A1 A2
  constraint coincident P5 P1
  constraint vertical L27
  constraint vertical L22.end A3.centre
  constraint coincident L22 A9.start
  constraint coincident L23 A9.end
  constraint coincident A3 A9.end
  constraint coincident A3.centre A9.centre
  constraint coincident P7 P6
  constraint vertical L42
  constraint vertical A20.centre L36.start
  constraint coincident L44.start L38
  constraint coincident L43.end L36
  constraint coincident L43.end A20
  constraint coincident A20.centre A26.centre
  constraint coincident P9 P8
  constraint vertical L54
  constraint vertical A32.centre L48.start
  constraint coincident L56.start L50
  constraint coincident L55.end L48
  constraint coincident L55.end A32
  constraint coincident A32.centre A38.centre
  constraint horizontal L58
  constraint vertical L59
  constraint horizontal L60
  constraint vertical L61
  constraint midpoint L21 P4
  measures "d221" distance of L15.start L15.end
  measures "d222" distance of L15.start L17.end
  measures "d223" vertical distance of L17.end P3
  measures "d224" horizontal distance of L17.end P3
  measures "d227" diameter of A0
  measures "d228" diameter of A1
  measures "d232" distance of P5 L27
  measures "d233" diameter of A3
  measures "d235" distance of L22.end A3.centre
  measures "d248" distance of P7 L42
  measures "d249" diameter of A20
  measures "d250" distance of A20.centre L36.start
  measures "d257" distance of P9 L54
  measures "d258" diameter of A32
  measures "d259" distance of A32.centre L48.start
  measures "d342" distance of L21.end L58.end
  measures "d343" distance of L21.start L58.end
hole "Hole2" at (0, 199.925, 34.3) at (0, 120, 34.3) at (0, 40.075, 34.3) direction (1, 0, 0) diameter 5 end up to surface (112.68 mm away) bodies 9
hole "Hole3" at (0, 40.075, 34.3) at (0, 120, 34.3) at (0, 199.925, 34.3) direction (1, 0, 0) diameter 5.4 end up to surface (107.12 mm away) bodies 7
hole "Hole4" at (-107.32, 199.925, 32.8) at (-107.32, 120, 32.8) at (-107.32, 40.075, 32.8) direction (-1, 0, 0) diameter 5 end up to surface (5.36 mm away) bodies 10
hole "Hole5" at (-107.32, 199.925, 32.8) at (-107.32, 120, 32.8) at (-107.32, 40.075, 32.8) direction (1, 0, 0) diameter 5.4 end up to surface (107.32 mm away) bodies 8
sketch "internal_nut_test_profile" plane through (0, 0, 0) normal (1, 0, 0) x (0, 0, -1)
  line L0 (-4.15, -2.396) -> (0, -4.792) construction
  line L1 (0, -4.792) -> (4.15, -2.396) construction
  line L2 (4.15, -2.396) -> (4.15, 2.396) construction
  line L3 (4.15, 2.396) -> (0, 4.792) construction
  line L4 (0, 4.792) -> (-4.15, 2.396) construction
  line L5 (-4.15, 2.396) -> (-4.15, -2.396) construction
  line L6 (0, 0) -> (0, 4.792) construction
  circle A0 centre (0, 4.592) radius 0.4 construction
  arc A1 (0.3989, 4.5617) -> (-0.3989, 4.5617) centre (0, 4.592) ccw
  arc A2 (-3.7511, 2.6263) -> (-4.15, 1.9354) centre (-3.9768, 2.296) ccw
  arc A3 (-4.15, -1.9354) -> (-3.7511, -2.6263) centre (-3.9768, -2.296) ccw
  arc A4 (-0.3989, -4.5617) -> (0.3989, -4.5617) centre (0, -4.592) ccw
  arc A5 (3.7511, -2.6263) -> (4.15, -1.9354) centre (3.9768, -2.296) ccw
  arc A6 (4.15, 1.9354) -> (3.7511, 2.6263) centre (3.9768, 2.296) ccw
  line L7 (-0.3989, 4.5617) -> (-3.7511, 2.6263)
  line L8 (-4.15, 1.9354) -> (-4.15, -1.9354)
  line L9 (-3.7511, -2.6263) -> (-0.3989, -4.5617)
  line L10 (0.3989, -4.5617) -> (3.7511, -2.6263)
  line L11 (4.15, -1.9354) -> (4.15, 1.9354)
  line L12 (3.7511, 2.6263) -> (0.3989, 4.5617)
  circle A7 centre (0, 0) radius 2.7
  line L13 (15, -15) -> (-15, -15)
  line L14 (-15, -15) -> (-15, 15)
  line L15 (-15, 15) -> (15, 15)
  line L16 (15, 15) -> (15, -15)
  line L17 (15, -15) -> (-15, 15) construction
  line L18 (-15, -15) -> (15, 15) construction
  dimension "d190" = 4.15
  dimension "d191" = 0.8
  dimension "d192" = 0.2
  dimension "d194" = 360
  dimension "d196" = 360
  dimension "d197" = 5.4
  dimension "d201" = 30
  constraint coincident L6.start A7.centre
  constraint vertical L5
  constraint coincident L6 A0.centre
  constraint coincident L4 A1.end
  constraint coincident L3 A1.start
  constraint coincident A0 A1.start
  constraint coincident A0.centre A1.centre
  constraint horizontal L13
  constraint perpendicular L13 L14
  constraint parallel L13 L15
  constraint parallel L14 L16
  constraint coincident L17 L6.start
  constraint coincident L18 L6.start
  constraint equal L14 L15
  measures "d190" distance of L6.start L5
  measures "d191" diameter of A0
  measures "d192" distance of L3.end A0.centre
  measures "d197" diameter of A7
  measures "d201" distance of L14.end L15.end
sketch "internal_nut_test_spacing" plane through (0, 0, 0) normal (0, 1, 0) x (1, 0, 0)
  line L0 (5, 15) -> (-5, 15)
  line L1 (-5, 15) -> (-5, -15)
  line L2 (-5, -15) -> (5, -15)
  line L3 (5, -15) -> (5, 15)
  line L4 (5, 15) -> (-5, -15) construction
  line L5 (-5, 15) -> (5, -15) construction
  line L6 (-1.75, -4.15) -> (1.75, -4.15)
  line L7 (1.75, -4.15) -> (1.75, 4.15)
  line L8 (1.75, 4.15) -> (-1.75, 4.15)
  line L9 (-1.75, 4.15) -> (-1.75, -4.15)
  line L10 (-1.75, -4.15) -> (1.75, 4.15) construction
  line L11 (1.75, -4.15) -> (-1.75, 4.15) construction
  line L12 (1.75, -4.15) -> (1.95, -4.15)
  line L13 (1.95, -4.15) -> (1.95, 4.15)
  line L14 (1.95, 4.15) -> (1.75, 4.15)
  point P0 (0, -4.15)
  dimension "d198" = 10
  dimension "d199" = 30
  dimension "d200" = 3.5
  dimension "d211" = 0.2
  constraint horizontal L0
  constraint perpendicular L0 L1
  constraint parallel L0 L2
  constraint parallel L1 L3
  constraint coincident L4 origin
  constraint coincident L5 origin
  constraint horizontal L6
  constraint perpendicular L6 L7
  constraint parallel L6 L8
  constraint parallel L7 L9
  constraint coincident L10 origin
  constraint coincident L11 origin
  constraint coincident L6 P0
  constraint horizontal L12
  constraint perpendicular L12 L13
  constraint perpendicular L7 L14
  measures "d198" distance of L1.end L2.end
  measures "d199" distance of L0.end L1.end
  measures "d200" distance of L7.end L8.end
  measures "d211" distance of L6.end L12.end
extrude "Extrude11" add sketch "internal_nut_test_profile" along normal up to surface (5 mm away) and the other way up to surface (5 mm away) separate body contours A1 A2 A3 A4 A5 A6 L7 L8 L9 L10 L11 L12 | L13 L14 L15 L16 makes body 11
extrude "Extrude12" cut sketch "internal_nut_test_profile" along normal up to surface (1.75 mm away) and the other way up to surface (1.75 mm away) contours A1 A2 A3 A4 A5 A6 L7 L8 L9 L10 L11 L12 bodies 11
extrude "Extrude13" add sketch "internal_nut_test_profile" along normal up to surface (0.2 mm away) from surface at 1.75 contours A7 bodies 11
sketch "internal nut spacing" plane through (0, 0, 0) normal (0, 1, 0) x (1, 0, 0)
  line L0 (112.68, 105.5) -> (112.68, -105.5)
  line L1 (-112.68, 105.5) -> (-112.68, -105.5)
  line L2 (112.68, -105.5) -> (-112.68, -105.5)
  line L3 (-112.68, -105.5) -> (-112.68, 105.5)
  line L4 (-112.68, 105.5) -> (112.68, 105.5)
  line L5 (112.68, 105.5) -> (112.68, -105.5)
  line L6 (100.68, -105.5) -> (100.68, 105.5)
  line L7 (-100.68, 105.5) -> (-100.68, -105.5)
  line L8 (101.68, -105.5) -> (101.68, 105.5)
  line L9 (105.18, 105.5) -> (105.18, -105.5)
  line L10 (107.12, -21.5) -> (107.12, -47.1)
  line L11 (-101.68, -105.5) -> (-101.68, 105.5)
  line L12 (-105.18, 105.5) -> (-105.18, -105.5)
  dimension "d215" = 12
  dimension "d216" = 12
  dimension "d217" = 1
  dimension "d218" = 3.5
  dimension "d219" = 1
  dimension "d220" = 3.5
  constraint horizontal L2
  constraint vertical L3
  constraint horizontal L4
  constraint vertical L5
  constraint coincident L1.start L3.end
  constraint coincident L0.end L2.start
  constraint coincident L2 L6.start
  constraint coincident L4 L6.end
  constraint perpendicular L4 L6
  constraint coincident L4 L7.start
  constraint coincident L2 L7.end
  constraint perpendicular L2 L7
  constraint coincident L2 L8.start
  constraint coincident L4 L8.end
  constraint perpendicular L4 L8
  constraint coincident L4 L9.start
  constraint coincident L2 L9.end
  constraint perpendicular L2 L9
  constraint coincident L2 L11.start
  constraint coincident L4 L11.end
  constraint perpendicular L4 L11
  constraint coincident L4 L12.start
  constraint coincident L2 L12.end
  constraint perpendicular L2 L12
  measures "d215" distance of L3 L7
  measures "d216" distance of L5 L6
  measures "d217" distance of L6.end L8.end
  measures "d218" distance of L8 L9
  measures "d219" distance of L7 L11
  measures "d220" distance of L11 L12
extrude "Extrude15" cut sketch "left_side_misc" along normal up to surface (3.5 mm away) from surface at 101.68 contours A9 A10 A11 A12 A13 A14 L28 L29 L30 L31 L32 L33 | L34 A15 A17 L35 A19 L37 A23 L39 A25 L43 L44 A26 | L46 A27 A29 L47 A31 L49 A35 L51 A37 L55 L56 A38 bodies 7
extrude "Extrude16" add sketch "left_side_misc" along normal blind 0.2 from surface at 105.18 contours A9 A10 A11 A12 A13 A14 L28 L29 L30 L31 L32 L33 | L34 A15 A17 L35 A19 L37 A23 L39 A25 L43 L44 A26 | L46 A27 A29 L47 A31 L49 A35 L51 A37 L55 L56 A38 bodies 7
extrude "Extrude17" cut sketch "right side panel" along normal up to surface (3.5 mm away) from surface at 2.14 contours A0 L55 L56 L57 A1 L59 A2 L62 L63 A4 A5 A6 | A7 A8 L67 L72 L75 L76 A9 A10 A12 L78 A13 L79 | A14 A15 L80 L85 L88 L89 A16 A17 A19 L91 A20 L92 bodies 8
extrude "Extrude18" add sketch "right side panel" against normal blind 0.2 from surface at 2.14 contours A0 L55 L56 L57 A1 L59 A2 L62 L63 A4 A5 A6 | A7 A8 L67 L72 L75 L76 A9 A10 A12 L78 A13 L79 | A14 A15 L80 L85 L88 L89 A16 A17 A19 L91 A20 L92 bodies 8
extrude "Extrude19" add sketch "right side panel" against normal blind 0.2 from surface at 22.04 contours A0 L55 L56 L57 A1 L59 A2 L62 L63 A4 A5 A6 | A7 A8 L67 L72 L75 L76 A9 A10 A12 L78 A13 L79 | A14 A15 L80 L85 L88 L89 A16 A17 A19 L91 A20 L92 bodies 8
extrude "Extrude20" add sketch "left_side_misc" along normal blind 0.2 from surface at 77.92 contours A9 A10 A11 A12 A13 A14 L28 L29 L30 L31 L32 L33 | L34 A15 A17 L35 A19 L37 A23 L39 A25 L43 L44 A26 | L46 A27 A29 L47 A31 L49 A35 L51 A37 L55 L56 A38 bodies 7